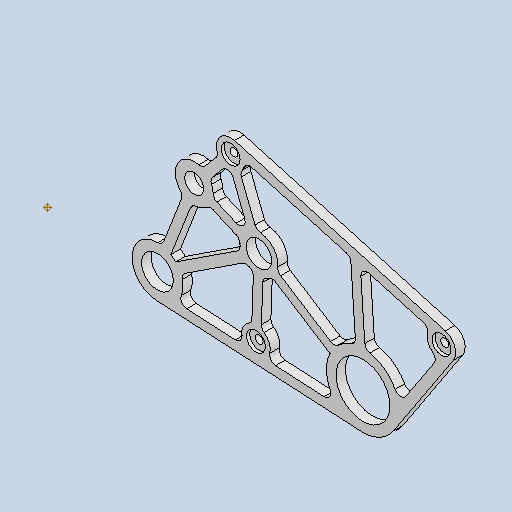
# Autodesk Inventor part: ギア抑え
Saved by Autodesk Inventor 2023 (Build 270158000, 158)
## iProperties
Created: 2022-01-29
Part Number: ギア抑え
Material: Aluminum 2014-T6
Document SubType Name: Modeling
Designer: acps
Density: 2.78927 g/cm^3
Appearance: Satin
Author: acps
Autodesk Inventor part; units mm, degrees
ref_plane "YZ Plane" through (0, 0, 0) normal (1, 0, 0) x (0, 1, 0)
ref_plane "XZ Plane" through (0, 0, 0) normal (0, 1, 0) x (-1, 0, 0)
ref_plane "XY Plane" through (0, 0, 0) normal (0, 0, 1) x (1, 0, 0)
sketch "Sketch4" plane through (0, 0, 0) normal (0, 0, 1) x (1, 0, 0)
  circle A0 centre (58.1571, 43.8132) radius 1.25
  circle A1 centre (46.616, 30) radius 3
  circle A2 centre (67.0906, 21) radius 4.025
  circle A3 centre (67.0906, 21) radius 6
  circle A4 centre (66.1789, -3.483) radius 1.25
  circle A5 centre (58.1571, 43.8132) radius 4.5
  circle A6 centre (66.1789, -3.483) radius 4.5
  circle A7 centre (46.616, 30) radius 6
  circle A8 centre (100, 0) radius 8.525
  circle A9 centre (124.8574, 25) radius 1.25
  circle A10 centre (124.8574, 25) radius 4.5
  circle A11 centre (100, 0) radius 11.525
  circle A12 centre (35, 0) radius 8.025
  line L0 (59.3787, 48.1442) -> (126.079, 29.331)
  line L1 (62.6476, 44.1052) -> (121.1813, 27.5954)
  line L2 (128.6167, 22.5266) -> (109.628, -6.3346)
  line L3 (123.7786, 20.6312) -> (111.3846, 1.7934)
  line L4 (100.7071, 11.5033) -> (99.1627, 33.8058)
  line L5 (97.7142, 11.2961) -> (96.0957, 34.6709)
  line L6 (71.181, 16.6104) -> (68.492, 18.3263) construction
  line L7 (72.7948, 19.1394) -> (91.174, 7.4113)
  line L8 (67.0906, 21) -> (100, 0) construction
  line L9 (67.0906, 21) -> (124.8574, 25) construction
  line L10 (105.9328, 11.9634) -> (90.1084, 10.8677) construction
  line L11 (100, 0) -> (97.4091, 37.4175) construction
  line L12 (65.705, -7.958) -> (65.6864, -7.956) construction
  line L13 (65.6967, -7.9837) -> (66.1849, -7.983) construction
  line L14 (65.3754, 15.2504) -> (65.4836, 18.1558) construction
  line L15 (67.8357, 0.7009) -> (68.3733, 15.1387)
  line L16 (67.0906, 21) -> (66.1789, -3.483) construction
  line L17 (68.492, 18.3263) -> (68.3733, 15.1387) construction
  line L18 (35, 0) -> (46.616, 30) construction
  line L19 (43.1196, 25.1241) -> (36.4478, 7.8933)
  line L20 (39.2454, 6.8101) -> (45.9172, 24.0408)
  line L21 (46.616, 30) -> (67.0906, 21) construction
  line L22 (51.3308, 26.289) -> (61.1686, 21.9646)
  line L23 (52.538, 29.0354) -> (59.937, 25.783)
  line L24 (61.1008, 40.4096) -> (66.369, 26.9565)
  line L25 (67.0906, 21) -> (58.1571, 43.8132) construction
  line L26 (58.3073, 39.3157) -> (62.6041, 28.3432)
  arc A13 (59.937, 25.783) -> (62.6041, 28.3432) centre (60.7418, 27.6139) ccw
  line L27 (62.6041, 28.3432) -> (63.5755, 25.8626) construction
  line L28 (59.937, 25.783) -> (62.3758, 24.711) construction
  line L29 (71.181, 16.6104) -> (89.5603, 4.8824)
  line L30 (68.3621, 14.8358) -> (68.492, 18.3263) construction
  line L31 (46.616, 30) -> (58.1571, 43.8132) construction
  line L32 (51.492, 33.4964) -> (56.5879, 39.5957)
  line L33 (49.1898, 35.4199) -> (54.2857, 41.5192)
  arc A14 (58.9156, 37.7626) -> (55.5184, 38.3156) centre (57.0532, 37.0333) ccw
  line L34 (35, 0) -> (67.0906, 21) construction
  line L35 (40.7753, 5.572) -> (61.4081, 19.074)
  line L36 (63.0508, 16.5638) -> (42.418, 3.0617)
  line L37 (65.3754, 15.2504) -> (64.8378, 0.8125)
  circle A15 centre (58.1571, 43.8132) radius 3
  circle A16 centre (124.8574, 25) radius 3
  circle A17 centre (66.1789, -3.483) radius 3
  line L38 (34.5679, -8.0134) -> (99.3794, -11.5083)
  line L39 (40.9773, -5.3546) -> (62.8723, -6.5353)
  line L40 (62.8723, -6.5353) -> (69.1381, -6.8732) construction
  line L41 (69.1381, -6.8732) -> (91.7966, -8.095)
  circle A18 centre (35, 0) radius 5.025
  point P0 (0, 0)
  point P1 (62.6167, 23.75)
  point P2 (63.8469, 21.7439)
  point P3 (63.7276, 4.995)
  point P4 (48.9428, 29.7841)
  point P5 (49.819, 30.1472)
  point P6 (62.9071, 26.3997)
  point P7 (50.9368, 32.3834)
  point P8 (50.8115, 33.0283)
  point P9 (57.8297, 40.9724)
  point P10 (62.9138, 26.4056)
  point P11 (67.612, 23.8643)
  point P12 (65.579, 26.356)
  point P13 (60.2796, 41.5397)
  point P14 (109.8309, 27.4562)
  point P15 (109.8687, 27.322)
  point P16 (93.5994, 9.6725)
  point P17 (91.8321, 9.416)
  point P18 (89.3299, 7.9976)
  point P19 (66.2271, 4.9132)
  point P20 (66.3467, 21.7081)
  point P21 (48.9379, 34.6835)
  point P22 (46.5685, 30.5773)
  point P23 (64.7751, 2.2487)
  point P24 (65.1323, 2.2448)
  point P25 (91.0705, 5.7078)
  point P26 (95.4376, 7.978)
  point P27 (111.7069, 25.6275)
  point P28 (110.5144, 29.861)
  point P29 (60.7307, 44.0105)
  point P30 (55.9361, 42.605)
  point P31 (92.4107, 6.1598)
  point P32 (92.438, 8.4126)
  point P33 (93.6914, 8.3068)
  point P34 (64.5533, 22.7819)
  point P35 (64.4718, 22.8265)
  point P36 (65.6711, 25.0181)
  point P37 (47.5045, 33.0609)
  point P38 (49.0002, 33.3514)
  point P39 (49.5268, 31.5741)
  point P40 (62.6167, 23.75)
  point P41 (63.8469, 21.7439)
  point P42 (63.7276, 4.995)
  point P43 (48.9428, 29.7841)
  point P44 (49.819, 30.1472)
  point P45 (62.9071, 26.3997)
  point P46 (50.9368, 32.3834)
  point P47 (50.8115, 33.0283)
  point P48 (57.8297, 40.9724)
  point P49 (62.9138, 26.4056)
  point P50 (67.612, 23.8643)
  point P51 (65.579, 26.356)
  point P52 (60.2796, 41.5397)
  point P53 (109.8309, 27.4562)
  point P54 (109.8687, 27.322)
  point P55 (93.5994, 9.6725)
  point P56 (91.8321, 9.416)
  point P57 (89.3299, 7.9976)
  point P58 (66.2271, 4.9132)
  point P59 (66.3467, 21.7081)
  point P60 (48.9379, 34.6835)
  point P61 (46.5685, 30.5773)
  point P62 (64.7751, 2.2487)
  point P63 (65.1323, 2.2448)
  point P64 (91.0705, 5.7078)
  point P65 (95.4376, 7.978)
  point P66 (111.7069, 25.6275)
  point P67 (110.5144, 29.861)
  point P68 (60.7307, 44.0105)
  point P69 (55.9361, 42.605)
  point P70 (92.4107, 6.1598)
  point P71 (92.438, 8.4126)
  point P72 (93.6914, 8.3068)
  point P73 (64.5533, 22.7819)
  point P74 (64.4718, 22.8265)
  point P75 (65.6711, 25.0181)
  point P76 (47.5045, 33.0609)
  point P77 (49.0002, 33.3514)
  point P78 (49.5268, 31.5741)
  point P79 (71.4365, 16.4474)
  point P80 (38.0841, 3.8109)
  point P81 (64.7982, -7.766)
  point P82 (66.607, -7.9626)
  dimension "d253" = 12
  dimension "d249" = 2.5
  dimension "d250" = 6
  dimension "d252" = 8.05
  dimension "d254" = 2.5
  dimension "d255" = 9
  dimension "d256" = 9
  dimension "d257" = 3
  dimension "d258" = 17.05
  dimension "d259" = 2.5
  dimension "d260" = 9
  dimension "d261" = 3
  dimension "d263" = 3
  dimension "d264" = 3
  dimension "d265" = 3
  dimension "d266" = 3
  dimension "d267" = 1.5
  dimension "d268" = 1.5
  dimension "d269" = 3
  dimension "d270" = 1.5
  dimension "d272" = 3
  dimension "d273" = 1.5
  dimension "d274" = 3
  dimension "d275" = 1.5
  dimension "d276" = 3
  dimension "d277" = 1.5
  dimension "d278" = 2
  dimension "d279" = 3
  dimension "d280" = 1.5
  dimension "d281" = 2
  dimension "d286" = 6
  dimension "d287" = 6
  dimension "d288" = 6
  dimension "d289" = 3
  dimension "d293" = 3
  dimension "d294" = 1.5
  dimension "d297" = 10.05
  dimension "d298" = 3
  constraints: 84 end point, 32 point on circle, 31 parallel, 17 centre point, 15 coincident, 13 tangent, 8 point on line, 2 perpendicular, 33 other
  measures "d249" diameter of A0
  measures "d250" diameter of A1
  measures "d252" diameter of A2
  measures "d254" diameter of A4
  measures "d255" diameter of A5
  measures "d256" diameter of A6
  measures "d257" radial gap between concentric circles of A1 A7
  measures "d258" diameter of A8
  measures "d259" diameter of A9
  measures "d260" diameter of A10
  measures "d263" distance between parallel lines of L1 L0
  measures "d264" distance between parallel lines of L2 L3
  measures "d265" distance between parallel lines of L4 L5
  measures "d266" distance between parallel lines of L6 L7
  measures "d267" distance between parallel lines of L7 L8
  measures "d268" distance between parallel lines of L11 L5
  measures "d269" distance between parallel lines of L14 L15
  measures "d270" distance between parallel lines of L14 L16
  measures "d272" distance between parallel lines of L19 L20
  measures "d273" distance between parallel lines of L18 L20
  measures "d274" distance between parallel lines of L22 L23
  measures "d275" distance between parallel lines of L22 L21
  measures "d276" distance between parallel lines of L26 L24
  measures "d277" distance between parallel lines of L24 L25
  measures "d278" radius of A13
  measures "d279" distance between parallel lines of L33 L32
  measures "d280" distance between parallel lines of L31 L32
  measures "d281" radius of A14
  measures "d286" diameter of A15
  measures "d287" diameter of A16
  measures "d288" diameter of A17
  measures "d289" distance between parallel lines of L38 L39
  measures "d293" distance between parallel lines of L35 L36
  measures "d294" distance between parallel lines of L36 L34
  measures "d297" diameter of A18
  measures "d298" radial gap between concentric circles of A18 A12
extrude "Extrusion3" add sketch "Sketch4" against normal blind 3 contours A3 | A3 L22 A7 L23 A13 L26 A5 L24 | L7 A11 L29 A3 | A5 | A11 | A3 L36 A12 L35 | A7 | L15 A6 L37 A3 | L5 L1 L4 A11 | A12 | L20 A12 L19 A7 | L32 A7 L33 A5 | A5 L0 A10 L1 | A6 | A11 L38 A12 L39 A6 L41 | L3 A10 L2 A11 | A10 | A15 | A16 | A17
extrude "Extrusion5" cut sketch "Sketch4" against normal blind 1 contours A15 | A16 | A17
fillet "Fillet4" radius 2 35 edges at (52.538, 29.0354, -1.5) (51.492, 33.4964, -1.5) (49.1898, 35.4199, -1.5) (54.2857, 41.5192, -1.5) (43.1196, 25.1241, -1.5) (36.4478, 7.8933, -1.5) (64.8378, 0.8125, -1.5) (62.8723, -6.5353, -1.5) (91.7966, -8.095, -1.5) (91.174, 7.4113, -1.5) (97.7142, 11.2961, -1.5) (72.7948, 19.1394, -1.5) (40.9773, -5.3546, -1.5) (42.418, 3.0617, -1.5) (66.369, 26.9565, -1.5) (100.7071, 11.5033, -1.5) (51.3308, 26.289, -1.5) (45.9172, 24.0408, -1.5) (61.1008, 40.4096, -1.5) (62.6476, 44.1052, -1.5) (56.5879, 39.5957, -1.5) (58.3073, 39.3157, -1.5) (96.0957, 34.6709, -1.5) (123.7786, 20.6312, -1.5) (121.1813, 27.5954, -1.5) (111.3846, 1.7934, -1.5) (99.1627, 33.8058, -1.5) (69.1381, -6.8732, -1.5) (67.8357, 0.7009, -1.5) (61.1686, 21.9646, -1.5) (61.4081, 19.074, -1.5) (65.3754, 15.2504, -1.5) (63.0508, 16.5638, -1.5) (68.3733, 15.1387, -1.5) (71.181, 16.6104, -1.5)
body "Solid2"
